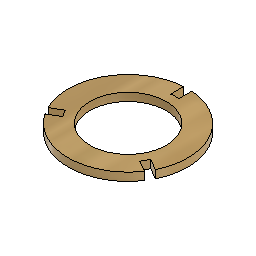
SPACER_LOWER (Autodesk Fusion 360 design; units mm, degrees)
Autodesk Fusion 360 part; units mm, degrees
sketch "Sketch1" plane through (0, 0, 0) normal (0, 0, 1) x (1, 0, 0)
  circle A0 centre (0, 0) radius 29.75
  circle A1 centre (0, 0) radius 18.925
  line L0 (0, 0) -> (0, 29.75) construction
  line L1 (-2, 23.3413) -> (2, 23.3413)
  line L2 (2, 23.3413) -> (2, 31)
  line L3 (2, 31) -> (-2, 31)
  line L4 (-2, 31) -> (-2, 23.3413)
  line L5 (-21.2141, -9.9386) -> (-27.8468, -13.7679)
  line L6 (-27.8468, -13.7679) -> (-25.8468, -17.2321)
  line L7 (-25.8468, -17.2321) -> (-19.2141, -13.4027)
  line L8 (-19.2141, -13.4027) -> (-21.2141, -9.9386)
  line L9 (19.2141, -13.4027) -> (25.8468, -17.2321)
  line L10 (25.8468, -17.2321) -> (27.8468, -13.7679)
  line L11 (27.8468, -13.7679) -> (21.2141, -9.9386)
  line L12 (21.2141, -9.9386) -> (19.2141, -13.4027)
  dimension "d1" = 59.5
  dimension "d78" = 37.85
  dimension "d128" = 360
  constraint coincident A0.centre A1.centre
  constraint coincident A0 L0.end
  constraint vertical L0
  constraint horizontal L1
  constraint vertical L2
  constraint horizontal L3
  constraint vertical L4
  measures "d1" diameter of A0
  measures "d78" diameter of A1
extrude "Extrude16" add sketch "Sketch1" along normal blind 4 contours A0 L1 L2 L4 L5 L7 L8 L9 L11 L12
